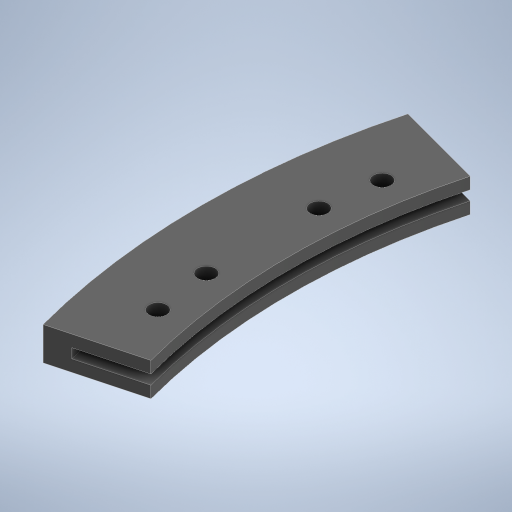
# Autodesk Inventor part: plate_cover
Saved by Autodesk Inventor 2024.1 (Build 281209000, 209)
## iProperties
Created: 2024-08-02
Part Number: plate_cover
Material: 一般
Document SubType Name: Modeling
Designer: hibik
Density: 1 g/cm^3
Appearance: 既定
Author: hibik
Autodesk Inventor part; units mm, degrees
ref_plane "YZ Plane" through (0, 0, 0) normal (1, 0, 0) x (0, 1, 0)
ref_plane "XZ Plane" through (0, 0, 0) normal (0, 1, 0) x (-1, 0, 0)
ref_plane "XY Plane" through (0, 0, 0) normal (0, 0, 1) x (1, 0, 0)
sketch "スケッチ1" plane through (0, 0, 0) normal (0, 1, 0) x (-1, 0, 0)
  circle A0 centre (0, 0) radius 105
  circle A1 centre (0, 0) radius 116
  line L0 (0, 0) -> (112.0474, 30.023)
  line L1 (0, 0) -> (112.0474, -30.023)
  line L2 (168, 0) -> (-168, 0) projected
  circle A2 centre (0, 0) radius 110 construction
  line L3 (0, 0) -> (108.3289, 19.1013) construction
  line L4 (109.5814, 9.5871) -> (0, 0) construction
  line L5 (109.5814, -9.5871) -> (0, 0) construction
  line L6 (0, 0) -> (108.3289, -19.1013) construction
  circle A3 centre (109.5814, 9.5871) radius 1.5
  circle A4 centre (108.3289, 19.1013) radius 1.5
  circle A5 centre (109.5814, -9.5871) radius 1.5
  circle A6 centre (108.3289, -19.1013) radius 1.5
  circle A7 centre (0, 0) radius 120
  line L7 (112.0474, 30.023) -> (115.9111, 31.0583)
  line L8 (112.0474, -30.023) -> (115.9111, -31.0583)
  point P0 (101.4222, -27.176)
  point P1 (101.4222, 27.176)
  dimension "d0" = 210
  dimension "d1" = 232
  dimension "d2" = 15
  dimension "d3" = 15
  dimension "d4" = 220
  dimension "d5" = 5
  dimension "d6" = 5
  dimension "d7" = 5
  dimension "d8" = 5
  dimension "d9" = 3
  dimension "d10" = 240
  constraints: 16 end point, 8 centre point, 8 point on circle, 7 coincident, 3 equal radius, 2 collinear
  measures "d0" diameter of A0
  measures "d1" diameter of A1
  measures "d2" angle of L2 L0
  measures "d3" angle of L2 L1
  measures "d4" diameter of A2
  measures "d5" angle of L2 L4
  measures "d6" angle of L3 L4
  measures "d7" angle of L5 L2
  measures "d8" angle of L6 L5
  measures "d9" diameter of A3
  measures "d10" diameter of A7
extrude "押し出し1" add sketch "スケッチ1" along normal blind 2 contours L2 A1 L1 A0 | A0 L0 A1 L2 | L2 A7 L8 A1 | A1 L7 A7 L2 picked at (107.2059, -25.9298) picked at (107.2059, 25.9298) picked at (115.3785, -27.3064) picked at (115.3785, 27.3064)
extrude "押し出し2" add sketch "スケッチ1" along normal blind 2.825 contours L2 A7 L8 A1 | A1 L7 A7 L2 picked at (115.3785, -27.3064) picked at (115.3785, 27.3064)
mirror "ミラー1" about plane through (-116.0237, 2.825, 0) normal (0, 1, 0)
equation "\"d6\" = d5"
equation "\"d7\" = d5"
equation "\"d8\" = d5"
